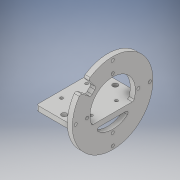
# Autodesk Inventor part: JeVois Camera Mount
Saved by Autodesk Inventor 2017 (Build 210142000, 142)
## iProperties
Created: 2018-02-07
Part Number: JeVois Camera Mount
Material: Generic
Document SubType Name: Modeling
Designer: 20franklinb
Density: 1 g/cm^3
Appearance: Default
Author: 20franklinb
Autodesk Inventor part; units mm, degrees
ref_plane "YZ Plane" through (0, 0, 0) normal (1, 0, 0) x (0, 1, 0)
sketch "Sketch1" plane through (0, 0, 0) normal (1, 0, 0) x (0, 1, 0)
  circle A0 centre (0, 0) radius 22.5
  circle A1 centre (0, 0) radius 40
  circle A2 centre (0, 36.75) radius 1.5
  circle A3 centre (0, 25.5) radius 1.5
  line L0 (0, 22.5) -> (0, 25.5)
  circle A4 centre (-36.75, 0) radius 1.5
  circle A5 centre (-25.5, 0) radius 1.5
  circle A6 centre (0, -36.75) radius 1.5
  circle A7 centre (0, -25.5) radius 1.5
  circle A8 centre (36.75, 0) radius 1.5
  circle A9 centre (25.5, 0) radius 1.5
  dimension "d0" = 45
  dimension "d9" = 80
  dimension "d12" = 3
  dimension "d13" = 3
  dimension "d64" = 3
  dimension "d67" = 360
  constraints: 9 centre point, 2 end point, 1 coincident, 1 vertical alignment, 19 other
  measures "d9" diameter of A1
  measures "d12" diameter of A2
  measures "d13" diameter of A3
  measures "d64" distance of L0.start L0.end
ref_plane "Work Plane1" through (5, 0, 0) normal (1, 0, 0) x (0, 0, -1)
sketch "Sketch2" plane through (5, 0, 0) normal (1, 0, 0) x (0, 0, -1)
  line L0 (0, 0) -> (0, -8.65)
  line L1 (0, -8.65) -> (23.4559, -8.65)
  line L2 (0, -8.65) -> (-23.4559, -8.65)
  line L3 (-23.4559, -8.65) -> (-30.4559, -8.65)
  line L4 (23.4559, -8.65) -> (30.4559, -8.65)
  line L5 (-30.4559, -8.65) -> (-30.4559, -13.65)
  line L6 (-30.4559, -13.65) -> (30.4559, -13.65)
  line L7 (30.4559, -13.65) -> (30.4559, -8.65)
  circle A0 centre (0, 0) radius 22.5
  dimension "d20" = 8.65
  dimension "d21" = 7
  dimension "d22" = 7
  dimension "d23" = 5
  dimension "d50" = 45
  constraints: 16 end point, 3 perpendicular, 2 horizontal, 2 vertical, 1 centre point, 1 coincident, 1 point on line
  measures "d20" distance of L0.start L0.end
  measures "d21" distance of L2.end L3.end
  measures "d22" distance of L1.end L4.end
  measures "d23" distance of L3.end L5.end
  measures "d50" diameter of A0
extrude "Extrusion2" add sketch "Sketch2" against normal blind 45 contours L1 A0 L6 L2 | L1 L4 L7 L6 A0 | A0 L6 L5 L3 L2
ref_plane "Work Plane2" through (5, -8.65, 23.4559) normal (0, 1, 0) x (1, 0, 0)
sketch "Sketch3" plane through (5, -8.65, 23.4559) normal (0, 1, 0) x (1, 0, 0)
  line L0 (-5, 23.4559) -> (-8.8, 23.4559)
  circle A0 centre (-8.8, 35.9559) radius 1.5
  circle A1 centre (-38.3, 35.9559) radius 1.5
  line L1 (-45, 53.9117) -> (-45, -7) projected
  circle A2 centre (-22.8, -1.9441) radius 2.5527
  circle A3 centre (-22.8, 48.8559) radius 2.5527
  line L2 (-8.8, 35.9559) -> (-38.3, 35.9559)
  line L3 (-8.8, 23.4559) -> (-8.8, 35.9559)
  line L4 (-8.8, 35.9559) -> (-8.8, 23.4559)
  circle A4 centre (-8.8, 10.9559) radius 1.5
  circle A5 centre (-38.3, 10.9559) radius 1.5
  line L5 (-8.8, 10.9559) -> (-38.3, 10.9559)
  line L6 (-8.8, 23.4559) -> (-8.8, 10.9559)
  dimension "d26" = 3.8
  dimension "d31" = 3
  dimension "d32" = 3
  dimension "d39" = 5.1054
  dimension "d40" = 5.1054
  dimension "d57" = 29.5
  dimension "d61" = 12.5
  constraints: 12 end point, 6 centre point, 4 symmetric about line, 2 horizontal, 1 perpendicular, 1 vertical, 2 other
  measures "d26" distance of L0.start L0.end
  measures "d31" diameter of A0
  measures "d32" diameter of A1
  measures "d39" diameter of A2
  measures "d40" diameter of A3
  measures "d57" distance of L2.start L2.end
  measures "d61" distance of L2.start L0.end
extrude "Extrusion3" cut sketch "Sketch3" against normal blind 50
extrude "Extrusion4" add sketch "Sketch1" along normal blind 5 contours A1 | A4 | A5 | A6 | A7 | A8 | A9
sketch "Sketch4" plane through (5, 0, 0) normal (1, 0, 0) x (0, 0, -1)
  circle A0 centre (0, 0) radius 40
  circle A1 centre (0, 0) radius 27
  line L0 (0, 0) -> (-31.9454, 24.0726)
  line L1 (-35, 0) -> (0, 0)
  line L2 (0, 0) -> (0, 35)
  line L3 (0, 0) -> (-24.0726, 31.9454)
  arc A2 (-16.249, 21.5632) -> (-21.5632, 16.249) centre (0, 0) ccw
  dimension "d51" = 54
  dimension "d53" = 37
  dimension "d54" = 37
  constraints: 8 end point, 6 point on circle, 3 centre point, 3 coincident, 2 point on line, 1 concentric, 1 horizontal, 1 perpendicular
  measures "d51" diameter of A1
  measures "d53" angle of L1 L0
  measures "d54" angle of L2 L3
extrude "Extrusion5" cut sketch "Sketch4" against normal blind 24.5 contours L3 A1 L0 A0 picked at (-25.4889, 24.8968)
fillet "Fillet1" radius 2 10 edges at (2.5, 31.9454, 24.0726) (2.5, 24.0726, 31.9454) (2.5, 16.249, 21.5632) (2.5, 21.5632, 16.249) (-40, -11.15, 30.4559) (-40, -11.15, -30.4559) (2.5, -8.65, -20.7708) (2.5, -8.65, 20.7708) (2.5, -13.65, 17.8865) (2.5, -13.65, -17.8865)
extrude "Extrusion6" cut sketch "Sketch1" along normal blind 24.5 contours A4 | A5 | A6 | A7 | A8 | A9
body "Solid1"
